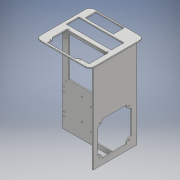
# Autodesk Inventor part: ExtrusionTray
Saved by Autodesk Inventor 2017 (Build 210142000, 142)
## iProperties
Created: 2019-06-19
Part Number: ExtrusionTray
Material: Generic
Document SubType Name: Modeling
Designer: DDeGo
Density: 1 g/cm^3
Appearance: Default
Author: DDeGo
Autodesk Inventor part; units mm, degrees
ref_plane "YZ Plane" through (0, 0, 0) normal (1, 0, 0) x (0, 1, 0)
ref_plane "XZ Plane" through (0, 0, 0) normal (0, 1, 0) x (-1, 0, 0)
ref_plane "XY Plane" through (0, 0, 0) normal (0, 0, 1) x (1, 0, 0)
sketch "Sketch1" plane through (0, 0, 0) normal (0, 0, 1) x (1, 0, 0)
  line L0 (15.5, 0) -> (174.5, 0)
  line L1 (190, 15.5) -> (190, 174.5)
  line L2 (174.5, 190) -> (15.5, 190)
  line L3 (0, 174.5) -> (0, 15.5)
  arc A0 (15.5, 190) -> (0, 174.5) centre (15.5, 174.5) ccw
  arc A1 (190, 174.5) -> (174.5, 190) centre (174.5, 174.5) ccw
  arc A2 (174.5, 0) -> (190, 15.5) centre (174.5, 15.5) ccw
  arc A3 (0, 15.5) -> (15.5, 0) centre (15.5, 15.5) ccw
  line L4 (15.5, 186.5) -> (174.5, 186.5) construction
  arc A4 (186.5, 174.5) -> (174.5, 186.5) centre (174.5, 174.5) ccw construction
  line L5 (186.5, 174.5) -> (186.5, 15.5) construction
  arc A5 (174.5, 3.5) -> (186.5, 15.5) centre (174.5, 15.5) ccw construction
  line L6 (174.5, 3.5) -> (15.5, 3.5) construction
  arc A6 (3.5, 15.5) -> (15.5, 3.5) centre (15.5, 15.5) ccw construction
  line L7 (3.5, 15.5) -> (3.5, 174.5) construction
  arc A7 (15.5, 186.5) -> (3.5, 174.5) centre (15.5, 174.5) ccw construction
  point P0 (0, 0)
  dimension "d75" = 12
  dimension "d76" = 183
  dimension "d77" = 3.5
  dimension "d78" = 183
  constraints: 16 end point, 16 point on circle, 8 centre point, 8 tangent, 4 parallel, 3 equal radius, 2 perpendicular, 2 point on line, 1 horizontal, 7 other
  measures "d75" radius of A7
  measures "d76" distance between parallel lines of L5 L7
  measures "d77" distance between parallel lines of L1 L5
  measures "d78" distance between parallel lines of L6 L4
extrude "Extrusion1" add sketch "Sketch1" along normal blind 4
sketch "Sketch2" plane through (0, 0, 0) normal (0, 0, -1) x (-1, 0, 0)
  line L0 (-186, 92) -> (-4, 92)
  line L1 (-4, 92) -> (-4, 89)
  line L2 (-4, 89) -> (-186, 89)
  line L3 (-186, 89) -> (-186, 92)
  line L4 (-174.5, 0) -> (-15.5, 0) projected
  line L5 (-190, 174.5) -> (-190, 15.5) projected
  line L6 (0, 15.5) -> (0, 174.5) projected
  point P0 (0, 0)
  dimension "d5" = 3
  dimension "d23" = 89
  dimension "d41" = 4
  dimension "d42" = 4
  constraints: 8 end point, 2 parallel, 1 horizontal, 1 perpendicular
  measures "d5" distance between parallel lines of L2 L0
  measures "d23" distance between parallel lines of L4 L2
  measures "d41" distance between parallel lines of L5 L3
  measures "d42" distance between parallel lines of L1 L6
extrude "Extrusion2" add sketch "Sketch2" along normal blind 170
sketch "Sketch3" plane through (0, 0, 4) normal (0, 0, 1) x (1, 0, 0)
  line L0 (25, 88.5) -> (175, 88.5) construction
  line L1 (175, 88.5) -> (175, 3.5) construction
  line L2 (175, 3.5) -> (25, 3.5) construction
  line L3 (25, 3.5) -> (25, 88.5) construction
  line L4 (31, 83.5) -> (169, 83.5) construction
  line L5 (169, 83.5) -> (169, 9.5) construction
  line L6 (145, 19.5) -> (31, 19.5) construction
  line L7 (31, 19.5) -> (31, 83.5) construction
  line L8 (145, 19.5) -> (145, 9.5) construction
  line L9 (145, 9.5) -> (169, 9.5) construction
  circle A0 centre (31, 83.5) radius 1.5
  circle A1 centre (31, 19.5) radius 1.5
  circle A2 centre (169, 83.5) radius 1.5
  circle A3 centre (145, 9.5) radius 1.5
  line L10 (34, 80.5) -> (34, 22.5) construction
  line L11 (34, 13.5) -> (142, 13.5) construction
  line L12 (173, 13.5) -> (173, 80.5)
  line L13 (173, 80.5) -> (34, 80.5)
  line L14 (15.5, 0) -> (174.5, 0) projected
  line L15 (190, 15.5) -> (190, 174.5) projected
  line L16 (34, 22.5) -> (27, 29.5)
  line L17 (27, 29.5) -> (27, 80.5)
  line L18 (27, 80.5) -> (34, 80.5)
  line L19 (34, 22.5) -> (34, 13.5)
  line L20 (142, 13.5) -> (134, 5.5)
  line L21 (134, 5.5) -> (34, 5.5)
  line L22 (34, 5.5) -> (34, 13.5)
  line L23 (142, 13.5) -> (173, 13.5)
  point P0 (0, 0)
  dimension "d8" = 3
  dimension "d9" = 138
  dimension "d10" = 64
  dimension "d11" = 74
  dimension "d12" = 114
  dimension "d13" = 6
  dimension "d14" = 6
  dimension "d15" = 5
  dimension "d16" = 6
  dimension "d17" = 8
  dimension "d18" = 2
  dimension "d19" = 4
  dimension "d20" = 9
  dimension "d24" = 85
  dimension "d26" = 15
  dimension "d40" = 3.5
  dimension "d79" = 135
  dimension "d80" = 2
  dimension "d81" = 3
  dimension "d82" = 135
  dimension "d83" = 3
  dimension "d84" = 2
  dimension "d85" = 88.5
  constraints: 44 end point, 7 parallel, 4 centre point, 4 coincident, 4 horizontal, 4 perpendicular, 3 equal radius, 3 vertical
  measures "d8" diameter of A0
  measures "d9" distance of L4.start L4.end
  measures "d10" distance of L6.end L4.start
  measures "d11" distance of L4.end L5.end
  measures "d12" distance of L6.start L6.end
  measures "d13" distance between parallel lines of L3 L7
  measures "d14" distance between parallel lines of L1 L5
  measures "d15" distance between parallel lines of L0 L4
  measures "d16" distance between parallel lines of L9 L2
  measures "d17" distance between parallel lines of L0 L13
  measures "d18" distance between parallel lines of L1 L12
  measures "d19" distance between parallel lines of L9 L11
  measures "d20" distance between parallel lines of L3 L10
  measures "d24" distance of L2.end L0.start
  measures "d26" distance between parallel lines of L15 L1
  measures "d40" distance between parallel lines of L14 L2
  measures "d79" angle of L19 L16
  measures "d80" distance between parallel lines of L3 L17
  measures "d81" horizontal distance of L10.end A1.centre
  measures "d82" angle of L23 L20
  measures "d83" horizontal distance of L11.end L8.end
  measures "d84" distance between parallel lines of L2 L21
  measures "d85" distance between parallel lines of L14 L0
extrude "Extrusion3" cut sketch "Sketch3" against normal blind 198.25
sketch "Sketch4" plane through (4, 92, 0) normal (0, 1, 0) x (1, 0, 0)
  line L0 (170, 165.44) -> (170, 10.5) construction
  line L1 (170, 10.5) -> (12.52, 10.5) construction
  line L2 (12.52, 10.5) -> (12.52, 165.44) construction
  line L3 (12.52, 165.44) -> (170, 165.44) construction
  circle A0 centre (170, 10.5) radius 2
  circle A1 centre (170, 165.44) radius 2
  circle A2 centre (12.52, 165.44) radius 2
  circle A3 centre (12.52, 33.36) radius 2
  line L4 (0, 0) -> (182, 0) projected
  line L5 (0, 0) -> (0, 170) projected
  line L6 (182, 0) -> (182, 170) projected
  point P0 (-4, 0)
  point P1 (-3, 350)
  dimension "d28" = 154.94
  dimension "d29" = 22.86
  dimension "d30" = 4
  dimension "d32" = 10.5
  dimension "d37" = 157.48
  dimension "d38" = 12
  dimension "d39" = 12.52
  constraints: 8 end point, 4 centre point, 3 coincident, 3 equal radius, 3 parallel, 1 perpendicular, 1 point on line
  measures "d28" distance between parallel lines of L3 L1
  measures "d29" distance of L1.end A3.centre
  measures "d30" diameter of A1
  measures "d32" distance between parallel lines of L4 L1
  measures "d37" distance between parallel lines of L0 L2
  measures "d38" distance between parallel lines of L6 L0
  measures "d39" distance between parallel lines of L5 L2
extrude "Extrusion4" cut sketch "Sketch4" against normal blind 198.25
sketch "Sketch5" plane through (4, 89, 0) normal (0, -1, 0) x (1, 0, 0)
  line L0 (105, -170) -> (105, -260)
  line L1 (105, -260) -> (0, -260)
  line L2 (0, -260) -> (0, -170)
  line L3 (105, -170) -> (0, -170)
  line L4 (0, -170) -> (182, -170) projected
  point P0 (-4, 0)
  dimension "d43" = 105
  dimension "d117" = 90
  constraints: 8 end point, 2 perpendicular, 1 coincident, 1 point on line, 1 vertical
  measures "d43" distance between parallel lines of L0 L2
  measures "d117" distance of L0.start L0.end
extrude "Extrusion5" add sketch "Sketch5" against normal up to surface (3 mm away)
sketch "Sketch6" plane through (0, 0, 0) normal (0, 0, -1) x (-1, 0, 0)
  line L0 (-183, 170) -> (-186, 170)
  line L1 (-186, 170) -> (-186, 15)
  line L2 (-186, 15) -> (-183, 15)
  line L3 (-183, 15) -> (-183, 170)
  line L4 (-4, 89) -> (-4, 92) projected
  line L5 (-15.5, 190) -> (-174.5, 190) projected
  line L6 (-174.5, 0) -> (-15.5, 0) construction
  arc A0 (-15.5, 0) -> (0, 15.5) centre (-15.5, 15.5) ccw construction
  line L7 (0, 15.5) -> (0, 174.5) construction
  line L8 (-3.5, 174.5) -> (-3.5, 15.5) construction
  arc A1 (-15.5, 3.5) -> (-3.5, 15.5) centre (-15.5, 15.5) ccw construction
  line L9 (-15.5, 3.5) -> (-174.5, 3.5) construction
  line L10 (-109, 89) -> (-109, 92) projected
  line L11 (-186, 92) -> (-186, 89) projected
  point P0 (0, 0)
  dimension "d47" = 3
  dimension "d48" = 20
  dimension "d49" = 15
  constraints: 12 end point, 2 parallel, 2 point on circle, 1 centre point, 1 collinear, 1 horizontal, 1 perpendicular, 2 other
  measures "d47" distance between parallel lines of L3 L1
  measures "d48" distance between parallel lines of L5 L0
  measures "d49" distance between parallel lines of L6 L2
extrude "Extrusion6" add sketch "Sketch6" along normal blind 315
sketch "Sketch7" plane through (186, 92, 0) normal (1, 0, 0) x (0, 0, -1)
  line L0 (182.5, -54.5) -> (287.5, -54.5) construction
  line L1 (287.5, -54.5) -> (287.5, 50.5) construction
  line L2 (287.5, 50.5) -> (182.5, 50.5) construction
  line L3 (182.5, 50.5) -> (182.5, -54.5) construction
  circle A0 centre (182.5, -54.5) radius 2
  circle A1 centre (182.5, 50.5) radius 2
  circle A2 centre (287.5, 50.5) radius 2
  circle A3 centre (287.5, -54.5) radius 2
  line L4 (175, -62) -> (295, -62)
  line L5 (295, -62) -> (295, 58)
  line L6 (295, 58) -> (175, 58)
  line L7 (175, 58) -> (175, -62)
  arc A4 (192.5, -62) -> (175, -44.5) centre (175, -62) ccw
  arc A5 (175, 40.5) -> (192.5, 58) centre (175, 58) ccw
  arc A6 (277.5, 58) -> (295, 40.5) centre (295, 58) ccw
  arc A7 (295, -44.5) -> (277.5, -62) centre (295, -62) ccw
  line L8 (170, -3) -> (170, 0) projected
  line L9 (0, -77) -> (315, -77) projected
  point P0 (0, -92)
  dimension "d52" = 105
  dimension "d53" = 105
  dimension "d54" = 4
  dimension "d55" = 120
  dimension "d56" = 35
  dimension "d57" = 5
  dimension "d58" = 15
  constraints: 16 end point, 8 centre point, 8 coincident, 8 point on circle, 8 point on line, 6 equal radius, 4 parallel, 2 perpendicular, 1 horizontal, 3 other
  measures "d52" distance between parallel lines of L2 L0
  measures "d53" distance between parallel lines of L1 L3
  measures "d54" diameter of A0
  measures "d55" distance of L6.end L4.start
  measures "d56" diameter of A4
  measures "d57" distance between parallel lines of L7 L8
  measures "d58" distance between parallel lines of L9 L4
extrude "Extrusion7" cut sketch "Sketch7" against normal up to surface (3 mm away) contours A0 | A1 | A2 | A3 | A4 L7 A5 L6 A6 L5 A7 L4
sketch "Sketch8" plane through (4, 92, -260) normal (0, 1, 0) x (1, 0, 0)
  line L0 (182, 55) -> (0, 55)
  line L1 (0, 55) -> (0, 0)
  line L2 (105, 0) -> (105, 40)
  line L3 (105, 40) -> (182, 40)
  line L4 (182, 55) -> (182, 40)
  line L5 (0, 0) -> (105, 0) projected
  line L6 (105, -90) -> (105, 0) projected
  line L7 (105, 0) -> (0, 0)
  point P0 (-4, -260)
  dimension "d63" = 15
  constraints: 12 end point, 3 perpendicular, 1 horizontal, 1 vertical
  measures "d63" distance between parallel lines of L0 L3
extrude "Extrusion8" add sketch "Sketch8" against normal up to surface (3 mm away)
sketch "Sketch9" plane through (186, 92, -315) normal (0, 1, 0) x (1, 0, 0)
  line L0 (-110.28, -44.96) -> (-180, -44.96) construction
  line L1 (-180, -44.96) -> (-180, -144.56) construction
  line L2 (-180, -144.56) -> (-110.28, -144.56) construction
  line L3 (-110.28, -144.56) -> (-110.28, -44.96) construction
  line L4 (-114.28, -53.96) -> (-176, -53.96) construction
  line L5 (-176, -53.96) -> (-176, -130.56) construction
  line L6 (-176, -130.56) -> (-114.28, -130.56) construction
  line L7 (-114.28, -130.56) -> (-114.28, -53.96) construction
  circle A0 centre (-114.28, -53.96) radius 1.75
  circle A1 centre (-114.28, -130.56) radius 1.75
  circle A2 centre (-176, -130.56) radius 1.75
  circle A3 centre (-176, -53.96) radius 1.75
  circle A4 centre (-12, -149.56) radius 2 projected
  line L8 (-182, -315) -> (-182, 0) projected
  point P0 (-186, -315)
  point P1 (92, -315)
  point P2 (0, -315)
  point P3 (-77, -145)
  dimension "d64" = 61.72
  dimension "d65" = 76.6
  dimension "d66" = 9
  dimension "d67" = 4
  dimension "d68" = 4
  dimension "d69" = 14
  dimension "d70" = 3.5
  dimension "d73" = 5
  dimension "d120" = 2
  constraints: 16 end point, 4 centre point, 4 coincident, 4 parallel, 3 equal radius, 2 horizontal, 2 perpendicular, 1 other
  measures "d64" distance of L4.start L4.end
  measures "d65" distance of L4.end L5.end
  measures "d66" distance between parallel lines of L0 L4
  measures "d67" distance between parallel lines of L3 L7
  measures "d68" distance between parallel lines of L1 L5
  measures "d69" distance between parallel lines of L2 L6
  measures "d70" diameter of A0
  measures "d73" distance from line of A4.centre L2
  measures "d120" distance between parallel lines of L8 L1
extrude "Extrusion9" cut sketch "Sketch9" against normal blind 10 contours A0 | A1 | A2 | A3
sketch "Sketch10" plane through (0, 0, 4) normal (0, 0, 1) x (1, 0, 0)
  line L0 (11, 139.7) -> (170, 139.7)
  line L1 (170, 139.7) -> (170, 95)
  line L2 (170, 95) -> (11, 95)
  line L3 (11, 95) -> (11, 139.7)
  line L4 (174.5, 190) -> (15.5, 190) projected
  line L5 (190, 15.5) -> (190, 174.5) projected
  line L6 (183, 92) -> (4, 92) projected
  line L7 (125, 186) -> (25, 186)
  line L8 (25, 186) -> (25, 147.5)
  line L9 (25, 147.5) -> (125, 147.5)
  line L10 (125, 147.5) -> (125, 186)
  line L11 (0, 174.5) -> (0, 15.5) projected
  point P0 (0, 0)
  dimension "d100" = 44.7
  dimension "d101" = 159
  dimension "d102" = 3
  dimension "d103" = 20
  dimension "d106" = 100
  dimension "d107" = 38.5
  dimension "d108" = 4
  dimension "d119" = 25
  constraints: 16 end point, 4 parallel, 2 horizontal, 2 perpendicular
  measures "d100" distance of L0.end L1.end
  measures "d101" distance between parallel lines of L3 L1
  measures "d102" distance between parallel lines of L6 L2
  measures "d103" distance between parallel lines of L1 L5
  measures "d106" distance between parallel lines of L8 L10
  measures "d107" distance between parallel lines of L7 L9
  measures "d108" distance between parallel lines of L4 L7
  measures "d119" distance between parallel lines of L11 L8
extrude "Extrusion10" cut sketch "Sketch10" against normal blind 10
sketch "Sketch11" plane through (186, 92, -315) normal (0, 1, 0) x (1, 0, 0)
  line L0 (-159.48, -300) -> (-22, -300)
  line L1 (-22, -300) -> (-22, -160)
  line L2 (-22, -160) -> (-159.48, -160)
  line L3 (-159.48, -160) -> (-159.48, -300)
  line L4 (-77, -145) -> (-3, -145) projected
  line L5 (-170.5, -315) -> (-11.5, -315) projected
  circle A0 centre (-169.48, -281.64) radius 2 projected
  circle A1 centre (-12, -304.5) radius 2 projected
  point P0 (-186, -315)
  point P1 (-90, -145)
  point P2 (-182, -145)
  point P3 (92, -145)
  dimension "d111" = 15
  dimension "d112" = 15
  dimension "d113" = 10
  dimension "d114" = 10
  constraints: 8 end point, 2 parallel, 1 horizontal, 1 perpendicular
  measures "d111" distance between parallel lines of L2 L4
  measures "d112" distance between parallel lines of L5 L0
  measures "d113" distance from line of A0.centre L3
  measures "d114" distance from line of A1.centre L1
extrude "Extrusion11" cut sketch "Sketch11" against normal blind 10 contours L3 L2 L1 L0
sketch "Sketch12" plane through (4, 89, 0) normal (0, -1, 0) x (1, 0, 0)
  line L0 (103.6, -317.44) -> (2, -317.44) construction
  line L1 (2, -317.44) -> (2, -170.44) construction
  line L2 (2, -170.44) -> (103.6, -170.44) construction
  line L3 (103.6, -170.44) -> (103.6, -317.44) construction
  line L4 (100.42, -276.16) -> (5.17, -276.16) construction
  line L5 (5.17, -276.16) -> (5.17, -199.96) construction
  line L6 (5.17, -199.96) -> (100.42, -199.96) construction
  line L7 (100.42, -199.96) -> (100.42, -276.16) construction
  circle A0 centre (100.42, -276.16) radius 1.75
  circle A1 centre (5.17, -276.16) radius 1.75
  circle A2 centre (100.42, -199.96) radius 1.75
  circle A3 centre (5.17, -199.96) radius 1.75
  line L8 (0, -315) -> (0, 0) projected
  circle A4 centre (12.52, -165.44) radius 2 projected
  point P0 (-4, 0)
  dimension "d121" = 101.6
  dimension "d122" = 147
  dimension "d123" = 3.5
  dimension "d124" = 95.25
  dimension "d125" = 76.2
  dimension "d126" = 41.28
  dimension "d127" = 3.18
  dimension "d128" = 2
  dimension "d129" = 5
  constraints: 16 end point, 4 centre point, 4 coincident, 4 parallel, 3 equal radius, 2 horizontal, 2 perpendicular
  measures "d121" distance of L0.start L0.end
  measures "d122" distance of L0.end L1.end
  measures "d123" diameter of A0
  measures "d124" distance of L5.end L6.end
  measures "d125" distance of L6.end L4.start
  measures "d126" distance between parallel lines of L0 L4
  measures "d127" distance between parallel lines of L3 L7
  measures "d128" distance between parallel lines of L8 L1
  measures "d129" distance from line of L2 A4.centre
extrude "Extrusion12" cut sketch "Sketch12" against normal blind 10 contours A0 | A1 | A2 | A3
body "Solid1"
